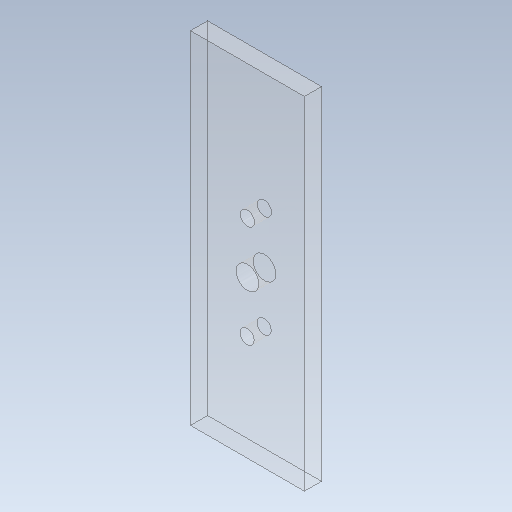
# Autodesk Inventor part: gard1
Saved by Autodesk Inventor 2021.1 (Build 251245010, 245A)
## iProperties
Created: 2023-11-23
Part Number: gard1
Material: PMMA Plastic
Document SubType Name: Modeling
Designer: M
Density: 1.188 g/cm^3
Appearance: Polycarbonate - Clear
Mass: 33.5762 g
Surface Area: 116.802 cm^2
Volume: 28.2628 cm^3
Author: M
Autodesk Inventor part; units mm, degrees
ref_plane "YZ Plane" through (0, 0, 0) normal (1, 0, 0) x (0, 1, 0)
ref_plane "XZ Plane" through (0, 0, 0) normal (0, 1, 0) x (-1, 0, 0)
ref_plane "XY Plane" through (0, 0, 0) normal (0, 0, 1) x (1, 0, 0)
sketch "Sketch1" plane through (0, 0, 0) normal (0, 0, 1) x (1, 0, 0)
  circle A0 centre (-0.1245, -8) radius 2.5
  circle A1 centre (-0.018, 28) radius 2.5
  line L0 (-20, 40) -> (-20, -45) projected
  line L1 (-20, -45) -> (20, -45) projected
  line L2 (20, -45) -> (20, 40) projected
  circle A2 centre (-0.1245, -8) radius 2.5 projected
  circle A3 centre (-0.018, 28) radius 2.5 projected
  line L3 (20, -45) -> (-20, -45)
  line L4 (-20, -45) -> (-20, 75)
  line L5 (-20, 75) -> (20, 75)
  line L6 (20, 75) -> (20, -45)
  circle A4 centre (0, 10) radius 4
  point P0 (0, 0)
  point P1 (20, 40)
  dimension "d0" = 120
  dimension "d1" = 8
  constraints: 8 end point, 3 centre point, 2 parallel, 1 horizontal, 1 perpendicular, 1 point on line
  measures "d0" distance of L3.end L4.end
  measures "d1" diameter of A4
extrude "Extrusion1" add sketch "Sketch1" along normal blind 6
body "Solid1"
